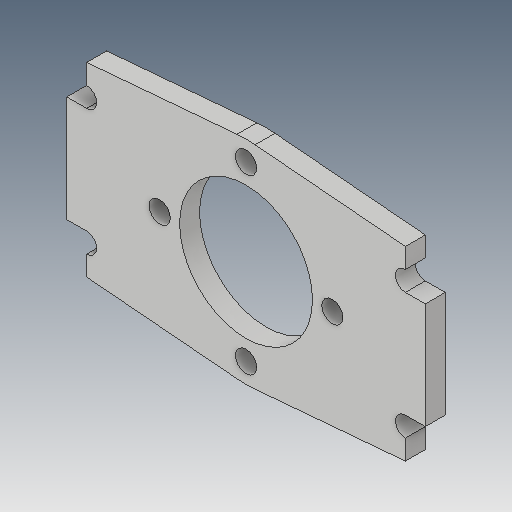
# Autodesk Inventor part: RS555-71K_MotorsupportAL
Saved by Autodesk Inventor 2019.4 (Build 234330000, 330)
## iProperties
Created: 2019-06-14
Part Number: RS555-71K_MotorsupportAL
Material: Generic
Document SubType Name: Modeling
Designer: AzLIer
Density: 1 g/cm^3
Appearance: Default
Mass: 3.53474 g
Surface Area: 31.7919 cm^2
Volume: 3.53474 cm^3
Author: AzLIer
Autodesk Inventor part; units mm, degrees
ref_plane "YZ Plane" through (0, 0, 0) normal (1, 0, 0) x (0, 1, 0)
ref_plane "XZ Plane" through (0, 0, 0) normal (0, 1, 0) x (-1, 0, 0)
ref_plane "XY Plane" through (0, 0, 0) normal (0, 0, 1) x (1, 0, 0)
sketch "スケッチ1" plane through (0, 0, 0) normal (0, 0, 1) x (1, 0, 0)
  circle A0 centre (0, 0) radius 10
  circle A1 centre (13, 0) radius 1.6
  circle A2 centre (0, 13) radius 1.6
  circle A3 centre (-13, 0) radius 1.6
  circle A4 centre (0, -13) radius 1.6
  circle A5 centre (0, 0) radius 16
  dimension "d0" = 20
  dimension "d1" = 3.2
  dimension "d2" = 13
  dimension "d5" = 360
  dimension "d7" = 6
  constraints: 6 centre point, 1 coincident, 1 horizontal alignment, 9 other
  measures "d0" diameter of A0
  measures "d1" diameter of A1
  measures "d2" distance of A1.centre point (0, 0)
  measures "d7" radial gap between concentric circles of A0 A5
extrude "押し出し1" add sketch "スケッチ1" along normal blind 3
sketch "スケッチ2" plane through (0, 0, 0) normal (0, 0, -1) x (-1, 0, 0)
  line L0 (-27, 8) -> (-27, -8)
  line L1 (27, -8) -> (27, 8)
  circle A0 centre (0, 0) radius 16 projected
  line L2 (24, -8) -> (27, -8)
  line L3 (-27, -8) -> (-24, -8)
  line L4 (-24, 8) -> (-27, 8)
  line L5 (27, 8) -> (24, 8)
  line L6 (-24, 14) -> (-24, 11)
  line L7 (-24, -11) -> (-24, -14)
  line L8 (24, -14) -> (24, -11)
  line L9 (24, 11) -> (24, 14)
  line L10 (-24, -14) -> (-1.3675, -15.9415)
  line L11 (1.3675, -15.9415) -> (24, -14)
  line L12 (24, 14) -> (1.3675, 15.9415)
  line L13 (-1.3675, 15.9415) -> (-24, 14)
  circle A1 centre (0, 0) radius 16 projected
  arc A2 (24, -8) -> (24, -11) centre (24, -9.5) ccw
  arc A3 (24, 11) -> (24, 8) centre (24, 9.5) ccw
  arc A4 (-24, 8) -> (-24, 11) centre (-24, 9.5) ccw
  arc A5 (-24, -11) -> (-24, -8) centre (-24, -9.5) ccw
  point P0 (-27, 0)
  point P1 (27, 0)
  dimension "d10" = 54
  dimension "d11" = 16
  dimension "d13" = 48
  dimension "d14" = 28
  dimension "d17" = 3
  constraints: 28 end point, 12 point on circle, 10 parallel, 8 point on line, 5 equal length, 4 centre point, 4 horizontal alignment, 4 tangent, 3 equal radius, 2 horizontal, 2 midpoint, 2 perpendicular, 1 vertical
  measures "d10" distance of L1.start L0.end
  measures "d11" distance of L0.end L0.start
  measures "d13" distance of L7.end L8.start
  measures "d14" distance of L6.start L7.end
  measures "d17" diameter of A5
extrude "押し出し2" add sketch "スケッチ2" against normal blind 3 contours L4 A4 L6 L13 A0 L10 L7 A5 L3 L0 | L12 L9 A3 L5 L1 L2 A2 L8 L11 A0
